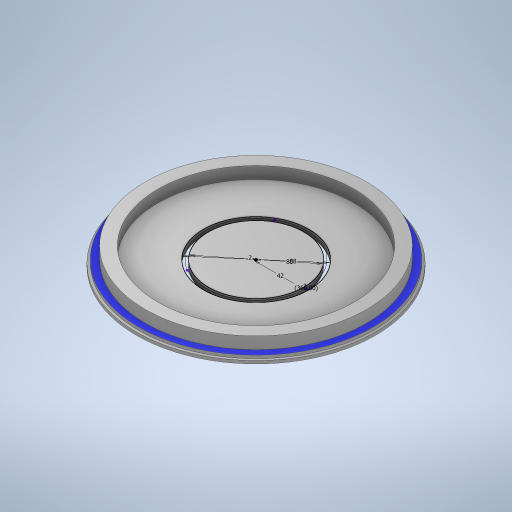
# Autodesk Inventor part: PlanetarygearboxBase
Saved by Autodesk Inventor 2024 (Build 280153000, 153)
## iProperties
Created: 2023-07-07
Part Number: PlanetarygearboxBase
Material: Generic
Document SubType Name: Modeling
Designer: westy
Density: 1 g/cm^3
Appearance: Anodized - Light Gray
Author: westy
Autodesk Inventor part; units mm, degrees
ref_plane "YZ Plane" through (0, 0, 0) normal (1, 0, 0) x (0, 1, 0)
ref_plane "XZ Plane" through (0, 0, 0) normal (0, 1, 0) x (-1, 0, 0)
ref_plane "XY Plane" through (0, 0, 0) normal (0, 0, 1) x (1, 0, 0)
sketch "Sketch1" plane through (0, 0, 0) normal (0, 1, 0) x (-1, 0, 0)
  circle A0 centre (0, 0) radius 100
  dimension "d0" = 200
  constraints: 1 centre point, 1 coincident
  measures "d0" diameter of A0
extrude "Extrusion1" add sketch "Sketch1" along normal blind 5
sketch "Sketch8" plane through (0, 5, 0) normal (0, 1, 0) x (1, 0, 0)
  circle A0 centre (0, 0) radius 1
  circle A1 centre (42, 0) radius 1
  circle A2 centre (-21, 36.3731) radius 1
  circle A3 centre (-21, -36.3731) radius 1
  circle A4 centre (0, 0) radius 44
  circle A5 centre (0, 0) radius 40
  point P0 (-20.5, -35.507)
  point P1 (-20.5, 35.507)
  point P2 (-21.5, 37.2391)
  point P3 (-21.5, -37.2391)
  point P4 (41, 0)
  point P5 (43, 0)
  dimension "d17" = 2
  dimension "d18" = 2
  dimension "d19" = 42
  dimension "d22" = 360
  dimension "d46" = 88
  dimension "d47" = 80
  constraints: 6 centre point, 3 coincident, 7 other
  measures "d17" diameter of A0
  measures "d18" diameter of A1
  measures "d19" distance of point (0, 0) A1.centre
  measures "d46" diameter of A4
  measures "d47" diameter of A5
sketch "Sketch9" plane through (0, 5, 0) normal (0, 1, 0) x (1, 0, 0)
  line L0 (80.8862, 2.8807) -> (72.2256, 0)
  line L1 (72.2256, 0) -> (80.8409, -3.9526)
  line L2 (80.3024, 10.1197) -> (71.9349, 6.4743)
  line L3 (71.9349, 6.4743) -> (80.8698, 3.3098)
  line L4 (79.072, 17.2772) -> (71.0649, 12.8964)
  line L5 (71.0649, 12.8964) -> (80.2475, 10.5456)
  line L6 (77.2049, 24.2956) -> (69.6228, 19.2147)
  line L7 (69.6228, 19.2147) -> (78.9792, 17.6965)
  line L8 (74.7163, 31.1184) -> (67.6202, 25.3783)
  line L9 (67.6202, 25.3783) -> (77.0749, 24.7049)
  line L10 (71.6261, 37.6906) -> (65.0731, 31.3375)
  line L11 (65.0731, 31.3375) -> (74.5501, 31.5144)
  line L12 (67.9592, 43.9594) -> (62.002, 37.0445)
  line L13 (62.002, 37.0445) -> (71.4251, 38.0702)
  line L14 (63.7451, 49.8742) -> (58.4318, 42.4532)
  line L15 (58.4318, 42.4532) -> (67.725, 44.3194)
  line L16 (59.0178, 55.3875) -> (54.3911, 47.52)
  line L17 (54.3911, 47.52) -> (63.4796, 50.2118)
  line L18 (53.8153, 60.4549) -> (49.9124, 52.2043)
  line L19 (49.9124, 52.2043) -> (58.7231, 55.6999)
  line L20 (48.1795, 65.0355) -> (45.032, 56.4683)
  line L21 (45.032, 56.4683) -> (53.4938, 60.7396)
  line L22 (42.1558, 69.0924) -> (39.7889, 60.2776)
  line L23 (39.7889, 60.2776) -> (47.8338, 65.2902)
  line L24 (35.7927, 72.5931) -> (34.2255, 63.6016)
  line L25 (34.2255, 63.6016) -> (41.7886, 69.3151)
  line L26 (29.1415, 75.5093) -> (28.3865, 66.4135)
  line L27 (28.3865, 66.4135) -> (35.407, 72.782)
  line L28 (22.2555, 77.8175) -> (22.319, 68.6907)
  line L29 (22.319, 68.6907) -> (28.7404, 75.6629)
  line L30 (15.1904, 79.4992) -> (16.0717, 70.4148)
  line L31 (16.0717, 70.4148) -> (21.8423, 77.9345)
  line L32 (8.003, 80.5409) -> (9.6951, 71.572)
  line L33 (9.6951, 71.572) -> (14.7684, 79.5787)
  line L34 (0.7512, 80.934) -> (3.2404, 72.1529)
  line L35 (3.2404, 72.1529) -> (7.5755, 80.5822)
  line L36 (-6.5067, 80.6755) -> (-3.2404, 72.1529)
  line L37 (-3.2404, 72.1529) -> (0.3217, 80.9369)
  line L38 (-13.7122, 79.7675) -> (-9.6951, 71.572)
  line L39 (-9.6951, 71.572) -> (-6.9347, 80.6399)
  line L40 (-20.8073, 78.2172) -> (-16.0717, 70.4148)
  line L41 (-16.0717, 70.4148) -> (-14.1353, 79.6936)
  line L42 (-27.7349, 76.0372) -> (-22.319, 68.6907)
  line L43 (-22.319, 68.6907) -> (-21.2221, 78.1057)
  line L44 (-34.4392, 73.245) -> (-28.3865, 66.4135)
  line L45 (-28.3865, 66.4135) -> (-28.138, 75.8889)
  line L46 (-40.8661, 69.863) -> (-34.2255, 63.6016)
  line L47 (-34.2255, 63.6016) -> (-34.8273, 73.0612)
  line L48 (-46.9641, 65.9185) -> (-39.7889, 60.2776)
  line L49 (-39.7889, 60.2776) -> (-41.2363, 69.6452)
  line L50 (-52.6839, 61.4433) -> (-45.032, 56.4683)
  line L51 (-45.032, 56.4683) -> (-47.3132, 65.6684)
  line L52 (-57.9796, 56.4734) -> (-49.9124, 52.2043)
  line L53 (-49.9124, 52.2043) -> (-53.0092, 61.1629)
  line L54 (-62.8084, 51.0488) -> (-54.3911, 47.52)
  line L55 (-54.3911, 47.52) -> (-58.2784, 56.165)
  line L56 (-67.1315, 45.2132) -> (-58.4318, 42.4532)
  line L57 (-58.4318, 42.4532) -> (-63.0784, 50.7148)
  line L58 (-70.9142, 39.0136) -> (-62.002, 37.0445)
  line L59 (-62.002, 37.0445) -> (-67.3705, 44.8564)
  line L60 (-74.1258, 32.4998) -> (-65.0731, 31.3375)
  line L61 (-65.0731, 31.3375) -> (-71.1202, 38.6367)
  line L62 (-76.7407, 25.7244) -> (-67.6202, 25.3783)
  line L63 (-67.6202, 25.3783) -> (-74.2973, 32.106)
  line L64 (-78.7377, 18.7419) -> (-69.6228, 19.2147)
  line L65 (-69.6228, 19.2147) -> (-76.8761, 25.3168)
  line L66 (-80.1007, 11.6084) -> (-71.0649, 12.8964)
  line L67 (-71.0649, 12.8964) -> (-78.836, 18.3238)
  line L68 (-80.8188, 4.3815) -> (-71.9349, 6.4743)
  line L69 (-71.9349, 6.4743) -> (-80.1612, 11.1832)
  line L70 (-80.8862, -2.8807) -> (-72.2256, 0)
  line L71 (-72.2256, 0) -> (-80.8409, 3.9526)
  line L72 (-80.3024, -10.1197) -> (-71.9349, -6.4743)
  line L73 (-71.9349, -6.4743) -> (-80.8698, -3.3098)
  line L74 (-79.072, -17.2772) -> (-71.0649, -12.8964)
  line L75 (-71.0649, -12.8964) -> (-80.2475, -10.5456)
  line L76 (-77.2049, -24.2956) -> (-69.6228, -19.2147)
  line L77 (-69.6228, -19.2147) -> (-78.9792, -17.6965)
  line L78 (-74.7163, -31.1184) -> (-67.6202, -25.3783)
  line L79 (-67.6202, -25.3783) -> (-77.0749, -24.7049)
  line L80 (-71.6261, -37.6906) -> (-65.0731, -31.3375)
  line L81 (-65.0731, -31.3375) -> (-74.5501, -31.5144)
  line L82 (-67.9592, -43.9594) -> (-62.002, -37.0445)
  line L83 (-62.002, -37.0445) -> (-71.4251, -38.0702)
  line L84 (-63.7451, -49.8742) -> (-58.4318, -42.4532)
  line L85 (-58.4318, -42.4532) -> (-67.725, -44.3194)
  line L86 (-59.0178, -55.3875) -> (-54.3911, -47.52)
  line L87 (-54.3911, -47.52) -> (-63.4796, -50.2118)
  line L88 (-53.8153, -60.4549) -> (-49.9124, -52.2043)
  line L89 (-49.9124, -52.2043) -> (-58.7231, -55.6999)
  line L90 (-48.1795, -65.0355) -> (-45.032, -56.4683)
  line L91 (-45.032, -56.4683) -> (-53.4938, -60.7396)
  line L92 (-42.1558, -69.0924) -> (-39.7889, -60.2776)
  line L93 (-39.7889, -60.2776) -> (-47.8338, -65.2902)
  line L94 (-35.7927, -72.5931) -> (-34.2255, -63.6016)
  line L95 (-34.2255, -63.6016) -> (-41.7886, -69.3151)
  line L96 (-29.1415, -75.5093) -> (-28.3865, -66.4135)
  line L97 (-28.3865, -66.4135) -> (-35.407, -72.782)
  line L98 (-22.2555, -77.8175) -> (-22.319, -68.6907)
  line L99 (-22.319, -68.6907) -> (-28.7404, -75.6629)
  line L100 (-15.1904, -79.4992) -> (-16.0717, -70.4148)
  line L101 (-16.0717, -70.4148) -> (-21.8423, -77.9345)
  line L102 (-8.003, -80.5409) -> (-9.6951, -71.572)
  line L103 (-9.6951, -71.572) -> (-14.7684, -79.5787)
  line L104 (-0.7512, -80.934) -> (-3.2404, -72.1529)
  line L105 (-3.2404, -72.1529) -> (-7.5755, -80.5822)
  line L106 (6.5067, -80.6755) -> (3.2404, -72.1529)
  line L107 (3.2404, -72.1529) -> (-0.3217, -80.9369)
  line L108 (13.7122, -79.7675) -> (9.6951, -71.572)
  line L109 (9.6951, -71.572) -> (6.9347, -80.6399)
  line L110 (20.8073, -78.2172) -> (16.0717, -70.4148)
  line L111 (16.0717, -70.4148) -> (14.1353, -79.6936)
  line L112 (27.7349, -76.0372) -> (22.319, -68.6907)
  line L113 (22.319, -68.6907) -> (21.2221, -78.1057)
  line L114 (34.4392, -73.245) -> (28.3865, -66.4135)
  line L115 (28.3865, -66.4135) -> (28.138, -75.8889)
  line L116 (40.8661, -69.863) -> (34.2255, -63.6016)
  line L117 (34.2255, -63.6016) -> (34.8273, -73.0612)
  line L118 (46.9641, -65.9185) -> (39.7889, -60.2776)
  line L119 (39.7889, -60.2776) -> (41.2363, -69.6452)
  line L120 (52.6839, -61.4433) -> (45.032, -56.4683)
  line L121 (45.032, -56.4683) -> (47.3132, -65.6684)
  line L122 (57.9796, -56.4734) -> (49.9124, -52.2043)
  line L123 (49.9124, -52.2043) -> (53.0092, -61.1629)
  line L124 (62.8084, -51.0488) -> (54.3911, -47.52)
  line L125 (54.3911, -47.52) -> (58.2784, -56.165)
  line L126 (67.1315, -45.2132) -> (58.4318, -42.4532)
  line L127 (58.4318, -42.4532) -> (63.0784, -50.7148)
  line L128 (70.9142, -39.0136) -> (62.002, -37.0445)
  line L129 (62.002, -37.0445) -> (67.3705, -44.8564)
  line L130 (74.1258, -32.4998) -> (65.0731, -31.3375)
  line L131 (65.0731, -31.3375) -> (71.1202, -38.6367)
  line L132 (76.7407, -25.7244) -> (67.6202, -25.3783)
  line L133 (67.6202, -25.3783) -> (74.2973, -32.106)
  line L134 (78.7377, -18.7419) -> (69.6228, -19.2147)
  line L135 (69.6228, -19.2147) -> (76.8761, -25.3168)
  line L136 (80.1007, -11.6084) -> (71.0649, -12.8964)
  line L137 (71.0649, -12.8964) -> (78.836, -18.3238)
  line L138 (80.8188, -4.3815) -> (71.9349, -6.4743)
  line L139 (71.9349, -6.4743) -> (80.1612, -11.1832)
  circle A0 centre (0, 0) radius 92.5
  arc A1 (-20.8073, 78.2172) -> (-21.2221, 78.1057) centre (0, 0) ccw
  arc A2 (-27.7349, 76.0372) -> (-28.138, 75.8889) centre (0, 0) ccw
  arc A3 (-34.4392, 73.245) -> (-34.8273, 73.0612) centre (0, 0) ccw
  arc A4 (-40.8661, 69.863) -> (-41.2363, 69.6452) centre (0, 0) ccw
  arc A5 (-67.9592, -43.9594) -> (-67.725, -44.3194) centre (0, 0) ccw
  arc A6 (-48.1795, -65.0355) -> (-47.8338, -65.2902) centre (0, 0) ccw
  arc A7 (-42.1558, -69.0924) -> (-41.7886, -69.3151) centre (0, 0) ccw
  arc A8 (-35.7927, -72.5931) -> (-35.407, -72.782) centre (0, 0) ccw
  arc A9 (-29.1415, -75.5093) -> (-28.7404, -75.6629) centre (0, 0) ccw
  arc A10 (-22.2555, -77.8175) -> (-21.8423, -77.9345) centre (0, 0) ccw
  arc A11 (-15.1904, -79.4992) -> (-14.7684, -79.5787) centre (0, 0) ccw
  arc A12 (-8.003, -80.5409) -> (-7.5755, -80.5822) centre (0, 0) ccw
  arc A13 (-0.7512, -80.934) -> (-0.3217, -80.9369) centre (0, 0) ccw
  arc A14 (6.5067, -80.6755) -> (6.9347, -80.6399) centre (0, 0) ccw
  arc A15 (13.7122, -79.7675) -> (14.1353, -79.6936) centre (0, 0) ccw
  arc A16 (20.8073, -78.2172) -> (21.2221, -78.1057) centre (0, 0) ccw
  arc A17 (27.7349, -76.0372) -> (28.138, -75.8889) centre (0, 0) ccw
  arc A18 (34.4392, -73.245) -> (34.8273, -73.0612) centre (0, 0) ccw
  arc A19 (40.8661, -69.863) -> (41.2363, -69.6452) centre (0, 0) ccw
  arc A20 (46.9641, -65.9185) -> (47.3132, -65.6684) centre (0, 0) ccw
  arc A21 (57.9796, -56.4734) -> (58.2784, -56.165) centre (0, 0) ccw
  arc A22 (62.8084, -51.0488) -> (63.0784, -50.7148) centre (0, 0) ccw
  arc A23 (67.1315, -45.2132) -> (67.3705, -44.8564) centre (0, 0) ccw
  arc A24 (70.9142, -39.0136) -> (71.1202, -38.6367) centre (0, 0) ccw
  arc A25 (74.1258, -32.4998) -> (74.2973, -32.106) centre (0, 0) ccw
  arc A26 (76.7407, -25.7244) -> (76.8761, -25.3168) centre (0, 0) ccw
  arc A27 (78.7377, -18.7419) -> (78.836, -18.3238) centre (0, 0) ccw
  arc A28 (80.1007, -11.6084) -> (80.1612, -11.1832) centre (0, 0) ccw
  arc A29 (80.8188, -4.3815) -> (80.8409, -3.9526) centre (0, 0) ccw
  arc A30 (80.8862, 2.8807) -> (80.8698, 3.3098) centre (0, 0) ccw
  arc A31 (80.3024, 10.1197) -> (80.2475, 10.5456) centre (0, 0) ccw
  arc A32 (79.072, 17.2772) -> (78.9792, 17.6965) centre (0, 0) ccw
  arc A33 (77.2049, 24.2956) -> (77.0749, 24.7049) centre (0, 0) ccw
  arc A34 (74.7163, 31.1184) -> (74.5501, 31.5144) centre (0, 0) ccw
  arc A35 (71.6261, 37.6906) -> (71.4251, 38.0702) centre (0, 0) ccw
  arc A36 (67.9592, 43.9594) -> (67.725, 44.3194) centre (0, 0) ccw
  arc A37 (63.7451, 49.8742) -> (63.4796, 50.2118) centre (0, 0) ccw
  arc A38 (59.0178, 55.3875) -> (58.7231, 55.6999) centre (0, 0) ccw
  arc A39 (42.1558, 69.0924) -> (41.7886, 69.3151) centre (0, 0) ccw
  arc A40 (35.7927, 72.5931) -> (35.407, 72.782) centre (0, 0) ccw
  arc A41 (29.1415, 75.5093) -> (28.7404, 75.6629) centre (0, 0) ccw
  arc A42 (22.2555, 77.8175) -> (21.8423, 77.9345) centre (0, 0) ccw
  arc A43 (15.1904, 79.4992) -> (14.7684, 79.5787) centre (0, 0) ccw
  arc A44 (8.003, 80.5409) -> (7.5755, 80.5822) centre (0, 0) ccw
  arc A45 (0.7512, 80.934) -> (0.3217, 80.9369) centre (0, 0) ccw
  arc A46 (-6.5067, 80.6755) -> (-6.9347, 80.6399) centre (0, 0) ccw
  arc A47 (-13.7122, 79.7675) -> (-14.1353, 79.6936) centre (0, 0) ccw
  circle A48 centre (0, 0) radius 82
  dimension "d29" = 360
  dimension "d31" = 185
  dimension "d37" = 164
  constraints: 280 end point, 2 centre point, 1 coincident, 494 other
  measures "d31" diameter of A0
  measures "d37" diameter of A48
extrude "Extrusion4" add sketch "Sketch9" along normal blind 10
sketch "Sketch10" plane through (0, 0, 0) normal (1, 0, 0) x (0, 1, 0)
  line L0 (0, 100) -> (5, 100) projected
  line L1 (12.4688, 100) -> (2.4688, 100)
  line L2 (2.4688, 100) -> (2.4688, 98)
  line L3 (2.4688, 98) -> (12.4688, 98)
  line L4 (12.4688, 98) -> (12.4688, 100)
  line L5 (-2.4938, 0) -> (14.9625, 0) projected
  point P0 (0, 0)
  dimension "d34" = 2
  dimension "d35" = 10
  constraints: 8 end point, 2 parallel, 1 horizontal, 1 perpendicular, 1 point on line
  measures "d34" distance of L1.end L2.end
  measures "d35" distance of L2.end L3.end
revolve "Revolution2" cut sketch "Sketch10" angle 360 about axis through (0, -10, 0) along (0, 1, 0)
extrude "Extrusion5" cut sketch "Sketch8" against normal blind 5 contours A0
sketch "Sketch11" plane through (0, 0, 0) normal (0, -1, 0) x (1, 0, 0)
  circle A0 centre (0, 0) radius 90
  circle A1 centre (0, 0) radius 1 projected
  circle A2 centre (0, 0) radius 85
  dimension "d40" = 180
  dimension "d41" = 170
  constraints: 2 centre point, 2 coincident
  measures "d40" diameter of A0
  measures "d41" diameter of A2
extrude "Extrusion6" cut sketch "Sketch11" against normal blind 5 contours A0
extrude "Extrusion7" cut sketch "Sketch8" against normal blind 10 contours A1 | A2 | A3
extrude "Extrusion8" cut sketch "Sketch8" against normal blind 10 contours A4
body "Solid1"
